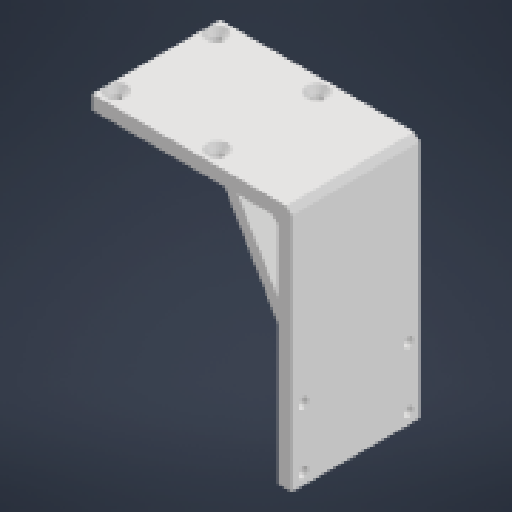
# Autodesk Inventor part: Kameraturm_Cognex_Halter
Saved by Autodesk Inventor 2026.1 (Build 301233020, 233B)
## iProperties
Created: 2025-10-16
Part Number: Kameraturm_Cognex_Halter
Material: Generisch
Document SubType Name: Modeling
Designer: iopeter
Density: 1 g/cm^3
Appearance: Vorgabe
Author: iopeter
Autodesk Inventor part; units mm, degrees
ref_plane "YZ Plane" through (0, 0, 0) normal (1, 0, 0) x (0, 1, 0)
ref_plane "XZ Plane" through (0, 0, 0) normal (0, 1, 0) x (-1, 0, 0)
ref_plane "XY Plane" through (0, 0, 0) normal (0, 0, 1) x (1, 0, 0)
sketch "Skizze1" plane through (0, 0, 0) normal (0, 0, 1) x (1, 0, 0)
  circle A0 centre (12.0667, -17.5) radius 2 projected
  circle A1 centre (12.0667, 17.5) radius 2 projected
  line L0 (17.0667, 22.5) -> (17.0667, -22.5) projected
  line L1 (7.0667, 22.5) -> (17.0667, 22.5) projected
  line L2 (7.0667, -22.5) -> (7.0667, 22.5) projected
  line L3 (17.0667, -22.5) -> (7.0667, -22.5) projected
  circle A2 centre (-23.4333, -17.5) radius 2 projected
  circle A3 centre (-23.4333, 17.5) radius 2 projected
  line L4 (-19.9333, 22.5) -> (-19.9333, -22.5) projected
  line L5 (-26.9333, 22.5) -> (-19.9333, 22.5) projected
  line L6 (-26.9333, -22.5) -> (-26.9333, 22.5) projected
  line L7 (-19.9333, -22.5) -> (-26.9333, -22.5) projected
  line L8 (43.2163, 19.557) -> (43.2163, 16.9277) projected
  line L9 (43.2163, -19.557) -> (43.2163, -16.9277) projected
  line L10 (43.2163, -20.3) -> (43.2163, -16.7) projected
  line L11 (43.2163, 20.3) -> (43.2163, 16.7) projected
  line L12 (-26.9333, 22.5) -> (43.2163, 22.5)
  line L13 (43.2163, 22.5) -> (43.2163, -22.5)
  line L14 (43.2163, -22.5) -> (-26.9333, -22.5)
  line L15 (-26.9333, -22.5) -> (-26.9333, 22.5)
  point P0 (0, 0)
  constraints: 8 end point, 2 parallel, 1 horizontal, 1 horizontal alignment, 1 perpendicular, 1 vertical alignment
extrude "Extrusion1" add sketch "Skizze1" along normal blind 5 contours A0 | A1 | L12 L13 L11 L8 L10 L9 L14 L0 | L0 L3 L2 L1 | L2 L14 L4 L12 | L4 L7 L6 L5 | A2 | A3
sketch "Skizze2" plane through (43.2163, -22.5, 0) normal (1, 0, 0) x (0, 0, -1)
  line L0 (0, 0) -> (-5, 0) projected
  line L1 (0, 0) -> (81.01, 0)
  line L2 (81.01, 0) -> (81.01, 45)
  line L3 (81.01, 45) -> (0, 45)
  line L4 (0, 45) -> (0, 0)
  circle A0 centre (77.01, 41) radius 1.8 construction
  circle A1 centre (77.01, 4) radius 1.8 construction
  arc A2 (54.796, 42.057) -> (57.124, 42.057) centre (55.96, 41) ccw construction
  arc A3 (57.124, 2.943) -> (54.796, 2.943) centre (55.96, 4) ccw construction
  circle A4 centre (55.96, 41) radius 1.75
  circle A5 centre (55.96, 4) radius 1.75
  circle A6 centre (77.01, 41) radius 1.75
  circle A7 centre (77.01, 4) radius 1.75
  point P0 (0, 22.5)
  dimension "d2" = 4
  dimension "d5" = 3.5
  dimension "d6" = 3.5
  dimension "d7" = 3.5
  dimension "d8" = 3.5
  constraints: 8 end point, 5 coincident, 4 centre point, 2 parallel, 1 horizontal, 1 perpendicular
  measures "d2" distance from line of L2 A1.centre
  measures "d5" diameter of A4
  measures "d6" diameter of A5
  measures "d7" diameter of A6
  measures "d8" diameter of A7
extrude "Extrusion2" add sketch "Skizze2" against normal blind 5
sketch "Skizze3" plane through (-26.9333, -22.5, 5) normal (0, -1, 0) x (1, 0, 0)
  line L0 (0, -5) -> (65.1497, -5) projected
  line L1 (31.7157, -5) -> (77.2703, -5) construction
  line L2 (65.1497, -86.01) -> (65.1497, -5) projected
  line L3 (51.1497, -5) -> (65.1497, -29.2487)
  line L4 (51.1497, -5) -> (79.1497, -5) construction
  line L5 (46.5308, -5) -> (65.1497, -37.2487)
  point P0 (26.9333, -5)
  dimension "d11" = 60
  dimension "d12" = 14
  dimension "d13" = 4
  constraints: 8 end point, 5 point on line, 2 horizontal, 1 equal length, 1 midpoint, 1 parallel
  measures "d11" angle of L3 L4
  measures "d12" distance of point (65.15, -5) L3.start
  measures "d13" distance between parallel lines of L3 L5
extrude "Extrusion3" add sketch "Skizze3" against normal up to surface (45 mm away) contours L0 L3 L2 L5
chamfer "Fasen1" distance 2 angle 45 2 edges at (38.2163, 0, 0) (43.2163, 0, 5)
sketch "Skizze4" plane through (0, 0, 5) normal (0, 0, 1) x (1, 0, 0)
  circle A0 centre (12.0667, 17.5) radius 2 projected
  circle A1 centre (12.0667, -17.5) radius 2 projected
  circle A2 centre (-23.4333, -17.5) radius 2 projected
  circle A3 centre (-23.4333, 17.5) radius 2 projected
  point P0 (0, 0)
hole "Bohrung1" at (12.0667, 17.5, 5) at (12.0667, -17.5, 5) at (-23.4333, -17.5, 5) at (-23.4333, 17.5, 5) direction (0, 0, -1) diameter 3.4 depth 8 countersink diameter 7.5 countersink angle 90 clearance for "Innensechskant-Senkkopfschraube DIN EN ISO 10642" size "M3" standard "DIN"
